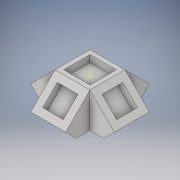
# Autodesk Inventor part: frame_nexus
Saved by Autodesk Inventor 2017 (Build 210142000, 142)
## iProperties
Created: 2017-01-19
Part Number: frame_nexus
Material: Generic
Document SubType Name: Modeling
Designer: Gabe Madonna
Density: 1 g/cm^3
Appearance: Default
Author: Gabe Madonna
Autodesk Inventor part; units mm, degrees
ref_plane "YZ Plane" through (0, 0, 0) normal (1, 0, 0) x (0, 1, 0)
ref_plane "XZ Plane" through (0, 0, 0) normal (0, 1, 0) x (-1, 0, 0)
ref_plane "XY Plane" through (0, 0, 0) normal (0, 0, 1) x (1, 0, 0)
sketch "Sketch1" plane through (0, 0, 0) normal (0, 1, 0) x (-1, 0, 0)
  point P0 (0, 0)
sketch "Sketch2" plane through (0, 0, 0) normal (0, 1, 0) x (-1, 0, 0)
  line L0 (9.525, -9.525) -> (-9.525, -9.525)
  line L1 (-9.525, -9.525) -> (-9.525, 9.525)
  line L2 (-9.525, 9.525) -> (9.525, 9.525)
  line L3 (9.525, 9.525) -> (9.525, -9.525)
  line L4 (-12.7, -12.7) -> (12.7, -12.7)
  line L5 (12.7, -12.7) -> (12.7, 12.7)
  line L6 (12.7, 12.7) -> (-12.7, 12.7)
  line L7 (-12.7, 12.7) -> (-12.7, -12.7)
  point P0 (0, 0)
  point P1 (0, 0)
  dimension "d0" = 19.05
  dimension "d1" = 3.175
  constraints: 16 end point, 1 coincident, 12 other
  measures "d0" distance of L2.end L0.start
  measures "d1" distance between parallel lines of L0 L4
extrude "Extrusion1" add sketch "Sketch2" along normal blind 5
sketch "Sketch3" plane through (0, 0, 0) normal (0, -1, 0) x (1, 0, 0)
  line L0 (12.7, -12.7) -> (-12.7, -12.7) projected
  line L1 (12.7, 12.7) -> (12.7, -12.7) projected
  line L2 (-12.7, 12.7) -> (12.7, 12.7) projected
  line L3 (-12.7, -12.7) -> (-12.7, 12.7) projected
  point P0 (0, 0)
extrude "Extrusion2" add sketch "Sketch3" along normal blind 20.4
sketch "Sketch4" plane through (12.7, 5, -12.7) normal (0, 0, -1) x (-1, 0, 0)
  line L0 (25.4, 0) -> (57.15, -31.75)
  line L1 (25.4, 0) -> (70.3013, 0) construction
  line L2 (25.4, -25.4) -> (25.4, 0) projected
  line L3 (25.4, -25.4) -> (50.8, -25.4)
  point P0 (12.7, -5)
  dimension "d6" = 45
  constraints: 6 end point, 2 horizontal, 1 equal length, 1 point on line
  measures "d6" angle of L0 L1
extrude "Extrusion3" add sketch "Sketch4" against normal up to surface (25.4 mm away)
sketch "Sketch5" plane through (-38.1, -20.4, -12.7) normal (-0.7071068, 0.7071068, 0) x (-0.7071068, -0.7071068, 0)
  line L0 (-35.921, 0) -> (-35.921, 25.4) projected
  line L1 (-35.921, 12.7) -> (-30.921, 12.7)
  line L2 (-30.921, 12.7) -> (-23.421, 12.7)
  line L3 (-30.921, 20.2) -> (-15.921, 20.2)
  line L4 (-15.921, 20.2) -> (-15.921, 5.2)
  line L5 (-15.921, 5.2) -> (-30.921, 5.2)
  line L6 (-30.921, 5.2) -> (-30.921, 20.2)
  point P0 (-41.3657, 12.7)
  dimension "d12" = 5
  dimension "d13" = 7.5
  constraints: 12 end point, 2 horizontal, 2 midpoint, 1 coincident, 9 other
  measures "d12" distance of L1.start L1.end
  measures "d13" distance of L1.end L2.end
extrude "Extrusion4" cut sketch "Sketch5" against normal blind 5
sketch "Sketch6" plane through (-38.1, -20.4, -12.7) normal (-0.7071068, 0.7071068, 0) x (-0.7071068, -0.7071068, 0)
  line L0 (-15.921, 20.2) -> (-15.921, 5.2) projected
  line L1 (-15.921, 12.7) -> (-10.921, 12.7)
  line L2 (-10.921, 12.7) -> (-10.921, 25.4)
  line L3 (-10.921, 25.4) -> (-10.921, 0)
  line L4 (-35.921, 0) -> (0, 0) projected
  line L5 (-10.921, 25.4) -> (0, 25.4)
  line L6 (0, 25.4) -> (0, 0)
  line L7 (0, 0) -> (-10.921, 0)
  line L8 (-10.921, 0) -> (-10.921, 25.4)
  point P0 (-41.3657, 12.7)
  point P1 (-17.9605, 0)
  dimension "d16" = 5
  constraints: 14 end point, 2 horizontal, 2 parallel, 2 point on line, 1 midpoint, 1 perpendicular, 1 vertical
  measures "d16" distance of L1.start L1.end
extrude "Extrusion5" cut sketch "Sketch6" against normal through all
pattern_circular "Circular Pattern2" count 4 over 360 about axis through (0, -10, 0) along (0, 1, 0) of "Extrusion5", "Extrusion4", "Extrusion3"
body "Solid1"
